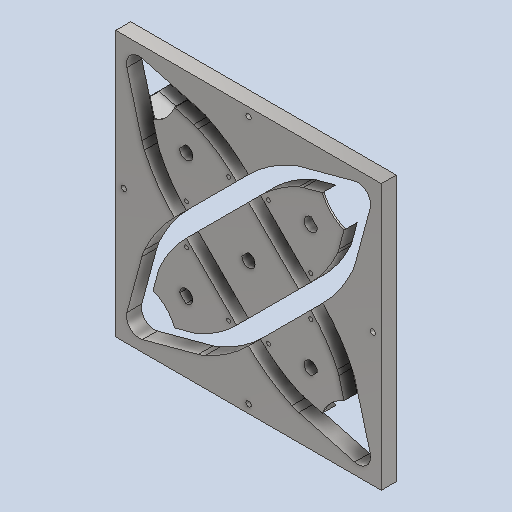
# Autodesk Inventor part: GuidePlateMetal
Saved by Autodesk Inventor 2022 (Build 260153000, 153)
## iProperties
Created: 2020-03-15
Part Number: GuidePlateMetal
Material: Generic
Document SubType Name: Modeling
Designer: elmar
Density: 1 g/cm^3
Appearance: Default
Author: elmar
Autodesk Inventor part; units mm, degrees
ref_plane "YZ Plane" through (0, 0, 0) normal (1, 0, 0) x (0, 1, 0)
ref_plane "XZ Plane" through (0, 0, 0) normal (0, 1, 0) x (-1, 0, 0)
sketch "Sketch41" plane through (0, 0, 0) normal (0, 0, 1) x (1, 0, 0)
  line L0 (80, -80) -> (-80, -80)
  line L1 (-80, -80) -> (-80, 80)
  line L2 (-80, 80) -> (80, 80)
  line L3 (80, 80) -> (80, -80)
  line L4 (80, -80) -> (-80, 80) construction
  line L5 (-80, -80) -> (80, 80) construction
  circle A0 centre (-37.5, 37.5) radius 37.5
  line L6 (0, -112) -> (0, 112) projected
  line L7 (-112, 0) -> (112, 0) projected
  circle A1 centre (-37.5, 37.5) radius 31.6165
  circle A2 centre (-37.5, 37.5) radius 21.4165
  circle A3 centre (37.5, -37.5) radius 31.6165
  circle A4 centre (37.5, -37.5) radius 21.4165
  line L8 (59.8562, -15.1438) -> (-15.1438, 59.8562)
  line L9 (52.6438, -22.3562) -> (-22.3562, 52.6438)
  line L10 (15.1438, -59.8562) -> (-59.8562, 15.1438)
  line L11 (22.3562, -52.6438) -> (-52.6438, 22.3562)
  circle A5 centre (-37.5, -37.5) radius 31.6165
  circle A6 centre (-37.5, -37.5) radius 21.4165
  circle A7 centre (37.5, 37.5) radius 31.6165
  circle A8 centre (37.5, 37.5) radius 21.4165
  line L12 (59.8562, 15.1438) -> (-15.1438, -59.8562)
  line L13 (52.6438, 22.3562) -> (-22.3562, -52.6438)
  line L14 (15.1438, 59.8562) -> (-59.8562, -15.1438)
  line L15 (22.3562, 52.6438) -> (-52.6438, -22.3562)
  line L16 (-37.5, 37.5) -> (-37.5, -37.5)
  circle A9 centre (-60.481, 60.481) radius 5
  line L17 (-49.8744, 49.8744) -> (-71.0876, 71.0876)
  arc A10 (-49.8744, 49.8744) -> (-71.0876, 71.0876) centre (-74.6231, 46.3388) ccw
  arc A11 (-71.0876, 71.0876) -> (-49.8744, 49.8744) centre (-46.3388, 74.6231) ccw
  arc A12 (-49.6403, 49.6403) -> (-71.3216, 71.3216) centre (-74.6231, 46.3388) ccw
  arc A13 (-71.3216, 71.3216) -> (-49.6403, 49.6403) centre (-46.3388, 74.6231) ccw
  line L18 (53.6853, -18.7098) -> (35.2271, 4.9396)
  circle A14 centre (44.4562, -6.8851) radius 5
  arc A15 (35.2271, 4.9396) -> (53.6853, -18.7098) centre (60.2225, 5.4203) ccw
  arc A16 (53.6853, -18.7098) -> (35.2271, 4.9396) centre (28.6899, -19.1906) ccw
  circle A17 centre (-37.5, 37.5) radius 17.5
  circle A18 centre (-37.5, 37.5) radius 7.5
  line L19 (-71.3216, 71.3216) -> (-49.6403, 49.6403)
  line L20 (-52.6438, 22.3562) -> (-59.8562, 15.1438)
  arc A19 (-62.7512, 26.1128) -> (-44.7125, 0) centre (17.6641, 62.3766) ccw
  arc A20 (-53.4529, 30.3059) -> (-37.5, 7.2125) centre (17.6641, 62.3766) ccw
  arc A21 (0, 44.7125) -> (-26.1128, 62.7512) centre (-62.3766, -17.6641) ccw
  arc A22 (-7.2125, 37.5) -> (-30.3059, 53.4529) centre (-62.3766, -17.6641) ccw
  line L21 (-37.5, 37.5) -> (-26.1128, 62.7512)
  circle A23 centre (-37.5, 37.5) radius 27.7
  circle A24 centre (-65.9013, 65.9013) radius 7.6655
  line L22 (-73.1417, 68.4185) -> (-44.18, 58.3498)
  line L23 (-73.5645, 66.0883) -> (-42.9116, 65.3403)
  line L24 (-73.038, 68.6991) -> (-44.4913, 57.5078)
  line L25 (-30.2936, 64.2462) -> (-63.9071, 73.3029)
  line L26 (-32.9472, 54.3974) -> (-44.4913, 57.5078)
  arc A25 (-60.0448, 43.663) -> (-44.4913, 57.5078) centre (-65.9013, 65.9013) ccw
  line L27 (-64.2462, 30.2936) -> (-73.3029, 63.9071)
  line L28 (-54.3974, 32.9472) -> (-57.5078, 44.4913)
  circle A26 centre (-37.5, 37.5) radius 4
  line L29 (-37.7505, 41.4921) -> (-41.4921, 37.7505)
  circle A27 centre (0, 0) radius 4
  line L30 (-0.2505, 3.9921) -> (-3.9921, 0.2505)
  point P0 (-37.5, 7.2125)
  point P1 (44.7125, 0)
  point P2 (-30.2875, 0)
  point P3 (-60.481, 60.481)
  dimension "d1039" = 35
  dimension "TrackWidth" = 10.2
  dimension "d715" = 160
  dimension "d718" = 75
  dimension "d721" = 10
  dimension "d722" = 30
  dimension "d723" = 0.2
  dimension "d1003" = 10
  dimension "d1004" = 30
  dimension "d1040" = 15
  dimension "d1487" = 8
  dimension "d1488" = 3
  constraints: 58 end point, 36 point on circle, 19 centre point, 17 point on line, 15 symmetric about line, 11 tangent, 9 coincident, 5 equal length, 5 horizontal, 5 parallel, 4 midpoint, 3 equal radius, 3 perpendicular, 1 concentric, 62 other
  measures "d715" distance of L1.end L2.end
  measures "d718" diameter of A0
  measures "d721" diameter of A9
  measures "d722" distance of L17.end L17.start
  measures "d723" radial gap between concentric circles of A10 A12
  measures "d1003" diameter of A14
  measures "d1004" distance of L18.start L18.end
  measures "d1040" diameter of A18
  measures "d1487" diameter of A26
  measures "d1488" distance from line of A0.centre L29
extrude "Extrusion39" add sketch "Sketch41" along normal blind 8
sketch "Sketch42" plane through (0, 0, 0) normal (0, 0, -1) x (-1, 0, 0)
  circle A0 centre (37.5, 37.5) radius 31.6165 projected
  circle A1 centre (37.5, 37.5) radius 21.4165 projected
  line L0 (-59.8562, -15.1438) -> (15.1438, 59.8562) projected
  line L1 (-52.6438, -22.3562) -> (22.3562, 52.6438) projected
  line L2 (-59.8562, 15.1438) -> (15.1438, -59.8562) projected
  line L3 (-15.1438, 59.8562) -> (59.8562, -15.1438) projected
  line L4 (-22.3562, -52.6438) -> (52.6438, 22.3562) projected
  line L5 (-15.1438, -59.8562) -> (59.8562, 15.1438) projected
  line L6 (-22.3562, 52.6438) -> (52.6438, -22.3562) projected
  arc A2 (44.7125, 0) -> (62.7512, 26.1128) centre (-17.6641, 62.3766) ccw projected
  arc A3 (37.5, 7.2125) -> (53.4529, 30.3059) centre (-17.6641, 62.3766) ccw projected
  arc A4 (26.1128, 62.7512) -> (0, 44.7125) centre (62.3766, -17.6641) ccw projected
  arc A5 (30.3059, 53.4529) -> (7.2125, 37.5) centre (62.3766, -17.6641) ccw projected
  line L7 (32.9472, 54.3974) -> (44.4913, 57.5078) projected
  arc A6 (44.4913, 57.5078) -> (60.0448, 43.663) centre (65.9013, 65.9013) ccw projected
  line L8 (54.3974, 32.9472) -> (57.5078, 44.4913) projected
  line L9 (30.2936, 64.2462) -> (63.9071, 73.3029) projected
  line L10 (64.2462, 30.2936) -> (73.3029, 63.9071) projected
  circle A7 centre (65.9013, 65.9013) radius 7.6655 projected
  circle A8 centre (37.5, 37.5) radius 17.5 projected
  circle A9 centre (37.5, 37.5) radius 27.7 projected
  point P0 (0, 0)
  point P1 (-44.7125, 0)
  point P2 (-37.5, -7.2125)
  point P3 (37.5, 7.2125)
  point P4 (44.7125, 0)
  point P5 (5.9103, 36.1978)
  point P6 (38.8022, 5.9103)
  point P7 (36.1978, 5.9103)
  point P8 (-7.2125, -37.5)
  point P9 (0, -44.7125)
  point P10 (7.2125, 37.5)
  point P11 (0, 44.7125)
  point P12 (5.9103, 38.8022)
  point P13 (60.5726, 60.5726)
  point P14 (10.2177, 53.4775)
  point P15 (53.4775, 10.2177)
  point P16 (-7.2125, 37.5)
  point P17 (30.2875, 0)
  point P18 (44.7125, 0)
  point P19 (47.9316, 51.551)
  point P20 (51.551, 47.9316)
  point P21 (45.0106, 68.2115)
  point P22 (68.2115, 45.0106)
  point P23 (0, 44.7125)
extrude "Extrusion40" cut sketch "Sketch42" against normal through all contours A2 L3 A0 | A0 L3 L4 A9 A2 | L10 A9 L9 A0 | A0 L9 A7 L10 | A9 L4 A1 L1 | A7 | L4 L6 A0 | A0 L1 L3 A9 L4 | A3 A9 L4 | A9 A3 A1 L4 | L6 L1 A0 | A9 L3 | A1 A3 A8 L8 A6 | A4 A9 L1 L3 A0 | A0 L3 A4 | L3 A0 L1 L6 L0 | A0 L3 L1 | A9 A5 L1 | L1 A1 A5 A9 | A1 A6 A8 L7 A5 | A6 A8 picked at (49.9917, 49.5888)
ref_plane "Work Plane2" through (0, 0, 7) normal (0, 0, 1) x (1, 0, 0)
extrude "Extrusion73" cut sketch "Sketch41" along normal through all contours A26 L16 L21 | L21 L16 A26 L29
extrude "Extrusion74" cut sketch "Sketch41" along normal through all contours A27 L7 L6 | L6 L7 A27 | L7 A27 L30 L6 | L6 A27 L7
ref_plane "Work Plane3" through (-80, 80, 0) normal (0.7071068, 0.7071068, 0) x (0, 0, 1)
pattern_circular "Circular Pattern6" count 4 over 360 about axis through (0, 0, -10) along (0, 0, 1) of "Extrusion40", "Extrusion73"
ref_plane "Work Plane6" through (-37.5, 7.2125, 7) normal (0, 0, 1) x (0.7071068, -0.7071068, 0)
sketch "Sketch75" plane through (0, 0, 7) normal (0, 0, -1) x (-1, 0, 0)
  arc A0 (37.5, 7.2125) -> (53.4529, 30.3059) centre (-17.6641, 62.3766) ccw projected
  arc A1 (53.4529, 30.3059) -> (54.3974, 32.9472) centre (37.5, 37.5) ccw projected
  line L0 (54.3974, 32.9472) -> (57.5078, 44.4913) projected
  arc A2 (44.4913, 57.5078) -> (57.5078, 44.4913) centre (65.9013, 65.9013) ccw projected
  line L1 (44.4913, 57.5078) -> (32.9472, 54.3974) projected
  arc A3 (32.9472, 54.3974) -> (30.3059, 53.4529) centre (37.5, 37.5) ccw projected
  arc A4 (30.3059, 53.4529) -> (7.2125, 37.5) centre (62.3766, -17.6641) ccw projected
  line L2 (7.2125, 37.5) -> (37.5, 7.2125) projected
  line L3 (-112, -112) -> (112, 112) projected
  line L4 (14.4366, 31.6901) -> (37.2742, 54.5276)
  line L5 (37.2742, 54.5276) -> (43.0737, 56.0902)
  line L6 (43.0737, 56.0902) -> (44.4913, 57.5078)
  line L7 (37.5, 37.5) -> (22.3562, 22.3562) construction
  line L8 (37.5, 7.2125) -> (7.2125, 37.5) projected
  line L9 (33.9645, 41.0355) -> (18.8207, 25.8918)
  line L10 (25.8918, 18.8207) -> (41.0355, 33.9645)
  arc A5 (41.0355, 33.9645) -> (33.9645, 41.0355) centre (37.5, 37.5) ccw
  arc A6 (18.8207, 25.8918) -> (25.8918, 18.8207) centre (22.3562, 22.3562) ccw
  line L11 (14.4366, 31.6901) -> (19.5278, 26.5989)
  arc A7 (44.4913, 57.5078) -> (57.5078, 44.4913) centre (65.9013, 65.9013) ccw projected
  line L12 (31.6901, 14.4366) -> (54.5276, 37.2742)
  line L13 (54.5276, 37.2742) -> (56.0902, 43.0737)
  line L14 (56.0902, 43.0737) -> (57.5078, 44.4913)
  line L15 (31.6901, 14.4366) -> (26.5989, 19.5278)
  point P0 (0, 0)
  point P1 (57.5078, 44.4913)
  dimension "d1056" = 5
  dimension "d1057" = 1
  dimension "SpringTipGuideWidth" = 7.2
  dimension "d1059" = 1
  constraints: 24 end point, 5 symmetric about line, 4 parallel, 4 point on circle, 4 tangent, 3 point on line, 2 centre point, 1 midpoint, 1 perpendicular
  measures "d1056" radius of A5
  measures "d1057" distance between parallel lines of L5 L1
  measures "SpringTipGuideWidth" distance of L4.start L11.end
  measures "d1059" distance between parallel lines of L8 L11
extrude "Extrusion50" cut sketch "Sketch75" along normal up to surface (7 mm away) contours L10 A5 L3 A2 L14 L13 L12 L15 | A5 L9 L11 L4 L5 L6 A2 L3
sketch "Sketch79" plane through (0, 0, 7) normal (0, 0, -1) x (-1, 0, 0)
  line L0 (-30.2875, 0) -> (0, 30.2875) projected
  line L1 (0, 30.2875) -> (30.2875, 0) projected
  line L2 (30.2875, 0) -> (0, -30.2875) projected
  line L3 (0, -30.2875) -> (-30.2875, 0) projected
  line L4 (54.3974, -32.9472) -> (57.5078, -44.4913) projected
  arc A0 (57.5078, -44.4913) -> (44.4913, -57.5078) centre (65.9013, -65.9013) ccw projected
  line L5 (44.4913, -57.5078) -> (32.9472, -54.3974) projected
  arc A1 (30.3059, -53.4529) -> (32.9472, -54.3974) centre (37.5, -37.5) ccw projected
  arc A2 (7.2125, -37.5) -> (30.3059, -53.4529) centre (62.3766, 17.6641) ccw projected
  line L6 (7.2125, -37.5) -> (37.5, -7.2125) projected
  arc A3 (53.4529, -30.3059) -> (37.5, -7.2125) centre (-17.6641, -62.3766) ccw projected
  arc A4 (54.3974, -32.9472) -> (53.4529, -30.3059) centre (37.5, -37.5) ccw projected
  arc A5 (-44.4913, -57.5078) -> (-57.5078, -44.4913) centre (-65.9013, -65.9013) ccw projected
  line L7 (-57.5078, -44.4913) -> (-54.3974, -32.9472) projected
  arc A6 (-53.4529, -30.3059) -> (-54.3974, -32.9472) centre (-37.5, -37.5) ccw projected
  arc A7 (-37.5, -7.2125) -> (-53.4529, -30.3059) centre (17.6641, -62.3766) ccw projected
  line L8 (-37.5, -7.2125) -> (-7.2125, -37.5) projected
  arc A8 (-30.3059, -53.4529) -> (-7.2125, -37.5) centre (-62.3766, 17.6641) ccw projected
  arc A9 (-32.9472, -54.3974) -> (-30.3059, -53.4529) centre (-37.5, -37.5) ccw projected
  line L9 (-32.9472, -54.3974) -> (-44.4913, -57.5078) projected
  line L10 (56.0902, 43.0737) -> (57.5078, 44.4913) projected
  arc A10 (44.4913, 57.5078) -> (57.5078, 44.4913) centre (65.9013, 65.9013) ccw projected
  line L11 (44.4913, 57.5078) -> (43.0737, 56.0902) projected
  line L12 (43.0737, 56.0902) -> (37.2742, 54.5276) projected
  line L13 (37.2742, 54.5276) -> (14.4366, 31.6901) projected
  line L14 (14.4366, 31.6901) -> (19.5278, 26.5989) projected
  line L15 (19.5278, 26.5989) -> (33.9645, 41.0355) projected
  arc A11 (41.0355, 33.9645) -> (33.9645, 41.0355) centre (37.5, 37.5) ccw projected
  line L16 (41.0355, 33.9645) -> (26.5989, 19.5278) projected
  line L17 (26.5989, 19.5278) -> (31.6901, 14.4366) projected
  line L18 (31.6901, 14.4366) -> (54.5276, 37.2742) projected
  line L19 (54.5276, 37.2742) -> (56.0902, 43.0737) projected
  line L20 (57.5078, 44.4913) -> (54.3974, 32.9472) projected
  arc A12 (53.4529, 30.3059) -> (54.3974, 32.9472) centre (37.5, 37.5) ccw projected
  arc A13 (37.5, 7.2125) -> (53.4529, 30.3059) centre (-17.6641, 62.3766) ccw projected
  line L21 (37.5, 7.2125) -> (7.2125, 37.5) projected
  arc A14 (30.3059, 53.4529) -> (7.2125, 37.5) centre (62.3766, -17.6641) ccw projected
  arc A15 (32.9472, 54.3974) -> (30.3059, 53.4529) centre (37.5, 37.5) ccw projected
  line L22 (32.9472, 54.3974) -> (44.4913, 57.5078) projected
  arc A16 (0, 44.7125) -> (-26.1128, 62.7512) centre (-62.3766, -17.6641) ccw projected
  arc A17 (-26.1128, 62.7512) -> (-30.2936, 64.2462) centre (-37.5, 37.5) ccw projected
  line L23 (-30.2936, 64.2462) -> (-63.9071, 73.3029) projected
  arc A18 (-63.9071, 73.3029) -> (-73.3029, 63.9071) centre (-65.9013, 65.9013) ccw projected
  line L24 (-73.3029, 63.9071) -> (-64.2462, 30.2936) projected
  arc A19 (-64.2462, 30.2936) -> (-62.7512, 26.1128) centre (-37.5, 37.5) ccw projected
  arc A20 (-62.7512, 26.1128) -> (-44.7125, 0) centre (17.6641, 62.3766) ccw projected
  arc A21 (-44.7125, 0) -> (-62.7512, -26.1128) centre (17.6641, -62.3766) ccw projected
  arc A22 (-62.7512, -26.1128) -> (-64.2462, -30.2936) centre (-37.5, -37.5) ccw projected
  line L25 (-64.2462, -30.2936) -> (-73.3029, -63.9071) projected
  arc A23 (-73.3029, -63.9071) -> (-63.9071, -73.3029) centre (-65.9013, -65.9013) ccw projected
  line L26 (-63.9071, -73.3029) -> (-30.2936, -64.2462) projected
  arc A24 (-30.2936, -64.2462) -> (-26.1128, -62.7512) centre (-37.5, -37.5) ccw projected
  arc A25 (-26.1128, -62.7512) -> (0, -44.7125) centre (-62.3766, 17.6641) ccw projected
  arc A26 (0, -44.7125) -> (26.1128, -62.7512) centre (62.3766, 17.6641) ccw projected
  arc A27 (26.1128, -62.7512) -> (30.2936, -64.2462) centre (37.5, -37.5) ccw projected
  line L27 (30.2936, -64.2462) -> (63.9071, -73.3029) projected
  arc A28 (63.9071, -73.3029) -> (73.3029, -63.9071) centre (65.9013, -65.9013) ccw projected
  line L28 (73.3029, -63.9071) -> (64.2462, -30.2936) projected
  arc A29 (64.2462, -30.2936) -> (62.7512, -26.1128) centre (37.5, -37.5) ccw projected
  arc A30 (62.7512, -26.1128) -> (44.7125, 0) centre (-17.6641, -62.3766) ccw projected
  arc A31 (44.7125, 0) -> (62.7512, 26.1128) centre (-17.6641, 62.3766) ccw projected
  arc A32 (62.7512, 26.1128) -> (64.2462, 30.2936) centre (37.5, 37.5) ccw projected
  line L29 (64.2462, 30.2936) -> (73.3029, 63.9071) projected
  arc A33 (73.3029, 63.9071) -> (63.9071, 73.3029) centre (65.9013, 65.9013) ccw projected
  line L30 (63.9071, 73.3029) -> (30.2936, 64.2462) projected
  arc A34 (30.2936, 64.2462) -> (26.1128, 62.7512) centre (37.5, 37.5) ccw projected
  arc A35 (26.1128, 62.7512) -> (0, 44.7125) centre (62.3766, -17.6641) ccw projected
  line L31 (80, 80) -> (80, -80) projected
  line L32 (80, -80) -> (-80, -80) projected
  line L33 (-80, -80) -> (-80, 80) projected
  line L34 (-80, 80) -> (80, 80) projected
  line L35 (-54.3974, 32.9472) -> (-57.5078, 44.4913) projected
  arc A36 (-57.5078, 44.4913) -> (-44.4913, 57.5078) centre (-65.9013, 65.9013) ccw projected
  line L36 (-44.4913, 57.5078) -> (-32.9472, 54.3974) projected
  arc A37 (-30.3059, 53.4529) -> (-32.9472, 54.3974) centre (-37.5, 37.5) ccw projected
  arc A38 (-7.2125, 37.5) -> (-30.3059, 53.4529) centre (-62.3766, -17.6641) ccw projected
  line L37 (-7.2125, 37.5) -> (-37.5, 7.2125) projected
  arc A39 (-53.4529, 30.3059) -> (-37.5, 7.2125) centre (17.6641, 62.3766) ccw projected
  arc A40 (-54.3974, 32.9472) -> (-53.4529, 30.3059) centre (-37.5, 37.5) ccw projected
  line L38 (57.5599, 44.6849) -> (56.0006, 43.1255)
  line L39 (56.0006, 43.1255) -> (54.438, 37.326)
  line L40 (54.438, 37.326) -> (31.6901, 14.5781)
  line L41 (31.6901, 14.5781) -> (26.7403, 19.5278)
  line L42 (26.7403, 19.5278) -> (41.1062, 33.8938)
  arc A41 (41.1062, 33.8938) -> (33.8938, 41.1062) centre (37.5, 37.5) ccw
  line L43 (33.8938, 41.1062) -> (19.5278, 26.7403)
  line L44 (19.5278, 26.7403) -> (14.5781, 31.6901)
  line L45 (14.5781, 31.6901) -> (37.326, 54.438)
  line L46 (37.326, 54.438) -> (43.1255, 56.0006)
  line L47 (43.1255, 56.0006) -> (44.6849, 57.5599)
  line L48 (23.0414, 40.1534) -> (27.9912, 35.2037)
  line L49 (44.6849, 57.5599) -> (55.0263, 60.3463)
  line L50 (44.4913, 57.5078) -> (32.9472, 54.3974) projected
  line L51 (38.7997, 55.9117) -> (37.4678, 54.5797)
  line L52 (43.0737, 56.0902) -> (43.2672, 56.1423)
  line L53 (37.2742, 54.5276) -> (43.0737, 56.0902) projected
  line L54 (-112, -112) -> (112, 112) projected
  arc A42 (44.4913, 57.5078) -> (57.5078, 44.4913) centre (65.9013, 65.9013) ccw projected
  line L55 (40.1534, 23.0414) -> (35.2037, 27.9912)
  line L56 (57.5599, 44.6849) -> (60.3463, 55.0263)
  line L57 (55.9117, 38.7997) -> (54.5797, 37.4678)
  line L58 (56.0902, 43.0737) -> (56.1423, 43.2672)
  line L59 (33.8938, 41.1062) -> (41.7207, 48.9332)
  arc A43 (48.9332, 48.9332) -> (41.7207, 48.9332) centre (45.327, 45.327) ccw
  line L60 (41.1062, 33.8938) -> (48.9332, 41.7207)
  arc A44 (48.9332, 41.7207) -> (48.9332, 48.9332) centre (45.327, 45.327) ccw
  arc A45 (55.0263, 60.3463) -> (60.3463, 55.0263) centre (73.7283, 73.7283) ccw
  arc A46 (-41.4921, 37.7505) -> (-37.7505, 41.4921) centre (-37.5, 37.5) ccw projected
  line L61 (-37.7505, 41.4921) -> (-41.4921, 37.7505) projected
  line L62 (3.9921, 0.2505) -> (0.2505, 3.9921) projected
  arc A47 (0.2505, 3.9921) -> (3.9921, 0.2505) centre (0, 0) ccw projected
  line L63 (37.7505, -41.4921) -> (41.4921, -37.7505) projected
  arc A48 (41.4921, -37.7505) -> (37.7505, -41.4921) centre (37.5, -37.5) ccw projected
  arc A49 (37.7505, 41.4921) -> (41.4921, 37.7505) centre (37.5, 37.5) ccw projected
  line L64 (41.4921, 37.7505) -> (37.7505, 41.4921) projected
  line L65 (-41.4921, -37.7505) -> (-37.7505, -41.4921) projected
  arc A50 (-37.7505, -41.4921) -> (-41.4921, -37.7505) centre (-37.5, -37.5) ccw projected
  point P0 (49.6403, 49.6403)
  point P1 (57.4673, 57.4673)
  point P2 (35.2037, 27.9912)
  point P3 (41.1062, 41.1062)
  point P4 (56.1423, 43.2672)
  point P5 (55.0639, 39.6489)
  point P6 (54.5797, 37.4678)
  point P7 (39.6489, 55.0639)
  dimension "d1077" = 0.1
  dimension "d1078" = 12.069
  dimension "d1079" = 11.069
  dimension "d1083" = 1
  dimension "SpringMaxCompression" = 11.069
  constraints: 40 end point, 11 point on circle, 4 centre point, 4 collinear, 4 point on line, 2 tangent, 1 coincident, 1 concentric, 1 equal radius, 1 parallel, 1 perpendicular, 25 other
  measures "d1077" distance between parallel lines of L45 L13
  measures "d1078" distance between parallel lines of L48 L14
  measures "d1079" distance of point (57.467, 57.467) point (49.64, 49.64)
  measures "d1083" distance of point (49.64, 49.64) A43.start
  measures "SpringMaxCompression" distance of point (48.933, 48.933) point (41.106, 41.106)
extrude "Extrusion52" add sketch "Sketch79" along normal blind 7 separate body contours L38 L39 L40 L55 L42 L60 A44 L54 A10 | A10 L54 A45 L56 L38 | L47 L49 A45 L54 A10 | A10 L54 A43 L59 L43 L48 L45 L46 L47
sketch "Sketch80" plane through (-27.9912, 35.2037, 7) normal (0.7071068, -0.7071068, 0) x (-0.7071068, -0.7071068, 0)
  line L0 (-7, 7) -> (0, 0)
  line L1 (-7, 0) -> (-7, 7) projected
  line L2 (-7, 7) -> (0, 7) projected
  line L3 (0, 7) -> (0, 0) projected
  line L4 (0, 0) -> (-7, 0) projected
  line L5 (10.2, 0) -> (10.2, 7) projected
  line L6 (10.2, 7) -> (17.2, 7) projected
  line L7 (17.2, 7) -> (17.2, 0) projected
  line L8 (17.2, 0) -> (10.2, 0) projected
  circle A0 centre (-3.5, 3.5) radius 2.75
  line L9 (25.414, -1) -> (-15.214, -1) projected
  line L10 (-15.214, -1) -> (-15.214, 7) projected
  line L11 (-15.214, 7) -> (-7.1, 7) projected
  line L12 (-7.1, 7) -> (-7.1, 0) projected
  line L13 (-7.1, 0) -> (0.1, 0) projected
  line L14 (0.1, 0) -> (0.1, 7) projected
  line L15 (0.1, 7) -> (10.1, 7) projected
  line L16 (10.1, 7) -> (10.1, 0) projected
  line L17 (10.1, 0) -> (17.3, 0) projected
  line L18 (17.3, 0) -> (17.3, 7) projected
  line L19 (17.3, 7) -> (25.414, 7) projected
  line L20 (25.414, 7) -> (25.414, -1) projected
  line L21 (-63.3516, 7) -> (-25.543, 7) projected
  line L22 (-25.543, 7) -> (-25.543, -1) projected
  line L23 (-25.543, -1) -> (-63.3516, -1) projected
  line L24 (-63.3516, -1) -> (-63.3516, 7) projected
  line L25 (35.743, 7) -> (73.5516, 7) projected
  line L26 (73.5516, 7) -> (73.5516, -1) projected
  line L27 (73.5516, -1) -> (35.743, -1) projected
  line L28 (35.743, -1) -> (35.743, 7) projected
  point P0 (5.1, 7)
  dimension "d1092" = 5.5
  constraints: 2 end point, 1 centre point, 1 coincident, 1 midpoint
  measures "d1092" diameter of A0
sketch "Sketch81" plane through (0, 0, 0) normal (0, 0, 1) x (1, 0, 0)
  line L0 (-44.6849, 57.5599) -> (-43.1255, 56.0006) projected
  line L1 (-43.1255, 56.0006) -> (-37.326, 54.438) projected
  line L2 (-37.326, 54.438) -> (-23.0414, 40.1534) projected
  line L3 (-23.0414, 40.1534) -> (-27.9912, 35.2037) projected
  line L4 (-27.9912, 35.2037) -> (-41.7207, 48.9332) projected
  arc A0 (-41.7207, 48.9332) -> (-48.9332, 41.7207) centre (-45.327, 45.327) ccw projected
  line L5 (-48.9332, 41.7207) -> (-35.2037, 27.9912) projected
  line L6 (-35.2037, 27.9912) -> (-40.1534, 23.0414) projected
  line L7 (-40.1534, 23.0414) -> (-54.438, 37.326) projected
  line L8 (-54.438, 37.326) -> (-56.0006, 43.1255) projected
  line L9 (-56.0006, 43.1255) -> (-57.5599, 44.6849) projected
  line L10 (-57.5599, 44.6849) -> (-60.3463, 55.0263) projected
  line L11 (-55.0263, 60.3463) -> (-44.6849, 57.5599) projected
  line L12 (-25.5163, 37.6785) -> (-39.8009, 51.9631)
  arc A1 (-60.3463, 55.0263) -> (-55.0263, 60.3463) centre (-73.7283, 73.7283) ccw projected
  point P0 (0, 0)
  dimension "SpringTipHoleDepth" = 20.2014
  constraints: 3 end point, 1 midpoint, 1 parallel, 1 perpendicular
  measures "SpringTipHoleDepth" distance of L12.start L12.end
sweep "Sweep1" cut profiles "Sketch80" path "Sketch81" bodies 2 path curves L12 contours A0 L0 | L0 A0
mirror "Mirror7" about plane through (-80, 80, 0) normal (0.7071068, 0.7071068, 0) of "Sweep1" bodies 2
sketch "Sketch83" plane through (-31.6901, 14.4366, 0) normal (-0.7071068, 0.7071068, 0) x (-0.7071068, -0.7071068, 0)
  circle A0 centre (-3.6, 3.5) radius 2.75 projected
  circle A1 centre (-3.6, 3.5) radius 1.25
  point P0 (-12.2, 0)
  dimension "d1103" = 2.5
  constraints: 1 centre point, 1 coincident
  measures "d1103" diameter of A1
extrude "Extrusion54" add sketch "Sketch83" along normal blind 1 contours A1 bodies 1
mirror "Mirror8" about plane through (-80, 80, 0) normal (0.7071068, 0.7071068, 0) of "Extrusion54" bodies 1
sketch "Sketch84" plane through (-37.5, 7.2125, 0) normal (0, 0, -1) x (-0.7071068, 0.7071068, 0)
  arc A0 (21.4165, 16.4165) -> (21.4165, 26.4165) centre (21.4165, 21.4165) ccw projected
  line L0 (1, 16.4165) -> (21.4165, 16.4165) projected
  circle A1 centre (21.4165, 21.4165) radius 5
  line L1 (24.4165, 24.0623) -> (24.4165, 18.7708) projected
  arc A2 (24.4165, 24.0623) -> (24.4165, 18.7708) centre (21.4165, 21.4165) ccw projected
  point P0 (-31.6165, 21.4165)
  point P1 (21.4165, 26.4165)
  constraints: 1 coincident, 3 other
extrude "Extrusion55" add sketch "Sketch84" along normal blind 1 bodies 1
pattern_circular "Circular Pattern7" count 4 over 360 about axis through (0, 0, -10) along (0, 0, 1) of "Extrusion50", "Extrusion54", "Mirror8", "Extrusion55" bodies 1
sketch "Sketch101" plane through (0, 0, 0) normal (0, 0, -1) x (-1, 0, 0)
  line L0 (0, 30.2875) -> (-30.2875, 0) projected
  line L1 (-30.2875, 0) -> (0, -30.2875) projected
  line L2 (0, -30.2875) -> (30.2875, 0) projected
  line L3 (30.2875, 0) -> (0, 30.2875) projected
  arc A0 (0, 44.7125) -> (-26.1128, 62.7512) centre (-62.3766, -17.6641) ccw projected
  arc A1 (26.1128, 62.7512) -> (0, 44.7125) centre (62.3766, -17.6641) ccw projected
  arc A2 (30.2936, 64.2462) -> (26.1128, 62.7512) centre (37.5, 37.5) ccw projected
  line L4 (30.2936, 64.2462) -> (63.9071, 73.3029) projected
  arc A3 (73.3029, 63.9071) -> (63.9071, 73.3029) centre (65.9013, 65.9013) ccw projected
  line L5 (73.3029, 63.9071) -> (64.2462, 30.2936) projected
  arc A4 (62.7512, 26.1128) -> (64.2462, 30.2936) centre (37.5, 37.5) ccw projected
  arc A5 (44.7125, 0) -> (62.7512, 26.1128) centre (-17.6641, 62.3766) ccw projected
  arc A6 (62.7512, -26.1128) -> (44.7125, 0) centre (-17.6641, -62.3766) ccw projected
  arc A7 (64.2462, -30.2936) -> (62.7512, -26.1128) centre (37.5, -37.5) ccw projected
  line L6 (64.2462, -30.2936) -> (73.3029, -63.9071) projected
  arc A8 (63.9071, -73.3029) -> (73.3029, -63.9071) centre (65.9013, -65.9013) ccw projected
  line L7 (63.9071, -73.3029) -> (30.2936, -64.2462) projected
  arc A9 (26.1128, -62.7512) -> (30.2936, -64.2462) centre (37.5, -37.5) ccw projected
  arc A10 (0, -44.7125) -> (26.1128, -62.7512) centre (62.3766, 17.6641) ccw projected
  arc A11 (-26.1128, -62.7512) -> (0, -44.7125) centre (-62.3766, 17.6641) ccw projected
  arc A12 (-30.2936, -64.2462) -> (-26.1128, -62.7512) centre (-37.5, -37.5) ccw projected
  line L8 (-30.2936, -64.2462) -> (-63.9071, -73.3029) projected
  arc A13 (-73.3029, -63.9071) -> (-63.9071, -73.3029) centre (-65.9013, -65.9013) ccw projected
  line L9 (-73.3029, -63.9071) -> (-64.2462, -30.2936) projected
  arc A14 (-62.7512, -26.1128) -> (-64.2462, -30.2936) centre (-37.5, -37.5) ccw projected
  arc A15 (-44.7125, 0) -> (-62.7512, -26.1128) centre (17.6641, -62.3766) ccw projected
  arc A16 (-62.7512, 26.1128) -> (-44.7125, 0) centre (17.6641, 62.3766) ccw projected
  arc A17 (-64.2462, 30.2936) -> (-62.7512, 26.1128) centre (-37.5, 37.5) ccw projected
  line L10 (-64.2462, 30.2936) -> (-73.3029, 63.9071) projected
  arc A18 (-63.9071, 73.3029) -> (-73.3029, 63.9071) centre (-65.9013, 65.9013) ccw projected
  line L11 (-63.9071, 73.3029) -> (-30.2936, 64.2462) projected
  arc A19 (-26.1128, 62.7512) -> (-30.2936, 64.2462) centre (-37.5, 37.5) ccw projected
  line L12 (80, -80) -> (-80, -80) projected
  line L13 (80, 80) -> (80, -80) projected
  line L14 (-80, 80) -> (80, 80) projected
  line L15 (-80, -80) -> (-80, 80) projected
  arc A20 (0.2505, 3.9921) -> (3.9921, 0.2505) centre (0, 0) ccw projected
  line L16 (0.2505, 3.9921) -> (3.9921, 0.2505) projected
extrude "Extrusion60" add sketch "Sketch101" along normal blind 1 bodies 1
sketch "Sketch43" plane through (0, 0, -1) normal (0, 0, 1) x (1, 0, 0)
  line L0 (-75, -75) -> (75, -75)
  line L1 (75, -75) -> (75, 75)
  line L2 (75, 75) -> (-75, 75)
  line L3 (-75, 75) -> (-75, -75)
  line L4 (-75, -75) -> (75, 75) construction
  line L5 (75, -75) -> (-75, 75) construction
  line L6 (-80, 80) -> (80, 80) projected
  point P0 (0, 0)
  point P1 (0, 75)
  point P2 (-75, 0)
  point P3 (0, -75)
  point P4 (75, 0)
  point P5 (-80, -80)
  point P6 (80, -80)
  dimension "d1250" = 5
  constraints: 12 end point, 6 midpoint, 3 point on line, 2 parallel, 2 perpendicular, 1 horizontal
  measures "d1250" distance between parallel lines of L2 L6
hole "Hole6" at (0, 75, -1) at (-75, 0, -1) at (0, -75, -1) at (75, 0, -1) direction (0, 0, 1) diameter 3.2 end through all countersink diameter 6.3 countersink angle 90 bodies 1
sketch "Sketch96" plane through (0, 0, 0) normal (0, 0, -1) x (-1, 0, 0)
  line L0 (37.5, -7.2125) -> (7.2125, -37.5) projected
  arc A0 (53.4529, -30.3059) -> (37.5, -7.2125) centre (-17.6641, -62.3766) ccw projected
  arc A1 (54.3974, -32.9472) -> (53.4529, -30.3059) centre (37.5, -37.5) ccw projected
  line L1 (57.5078, -44.4913) -> (54.3974, -32.9472) projected
  arc A2 (57.5078, -44.4913) -> (44.4913, -57.5078) centre (65.9013, -65.9013) ccw projected
  line L2 (32.9472, -54.3974) -> (44.4913, -57.5078) projected
  arc A3 (30.3059, -53.4529) -> (32.9472, -54.3974) centre (37.5, -37.5) ccw projected
  arc A4 (7.2125, -37.5) -> (30.3059, -53.4529) centre (62.3766, 17.6641) ccw projected
  circle A5 centre (37.5, -37.5) radius 5 projected
  point P0 (0, 0)
extrude "Extrusion57" add sketch "Sketch96" along normal blind 1 separate body
sketch "Sketch99" plane through (0, 0, -1) normal (0, 0, -1) x (-1, 0, 0)
  line L0 (37.5, -7.2125) -> (7.2125, -37.5) projected
  arc A0 (53.4529, -30.3059) -> (37.5, -7.2125) centre (-17.6641, -62.3766) ccw projected
  arc A1 (7.2125, -37.5) -> (30.3059, -53.4529) centre (62.3766, 17.6641) ccw projected
  circle A2 centre (37.4468, -12.0033) radius 3.35
  circle A3 centre (12.0033, -37.4468) radius 3.35
  point P0 (0, 0)
  dimension "d1222" = 6.7
  dimension "d1482" = 2
  dimension "d1484" = 4
  dimension "d1485" = 2
  constraints: 4 tangent, 2 centre point, 1 equal radius
  measures "d1222" diameter of A2
hole "Hole11" at (-12.0033, -37.4468, -1) at (-37.4468, -12.0033, -1) direction (0, 0, 1) diameter 2.459 end through all countersink diameter 7 countersink angle 90 bodies 1
pattern_circular "Circular Pattern15" count 4 over 360 about axis through (0, 0, -10) along (0, 0, 1) of "Hole11" bodies 1 3
hole "Hole15" at (-37.4468, -12.0033, -1) at (-12.0033, -37.4468, -1) direction (0, 0, 1) diameter 3.2 end through all countersink diameter 7 countersink angle 90 bodies 3
sketch "Sketch132" plane through (0, 0, 0) normal (0, 0, -1) x (-1, 0, 0)
  line L0 (16.9008, 39.8111) -> (29.1532, 52.0634) projected
  arc A0 (30.047, 52.5803) -> (29.1532, 52.0634) centre (30.5674, 50.6492) ccw projected
  line L1 (30.047, 52.5803) -> (43.0737, 56.0902) projected
  line L2 (14.5583, 32.0946) -> (36.887, 54.4233)
  line L3 (37.326, 54.438) -> (23.0414, 40.1534) projected
  line L4 (14.5583, 32.0946) -> (16.4013, 38.9345)
  arc A1 (16.9182, 39.8284) -> (16.4013, 38.9345) centre (18.3324, 38.4142) ccw
  line L5 (14.5871, 32.2484) -> (16.3839, 38.9172) projected
  arc A2 (16.9008, 39.8111) -> (16.3839, 38.9172) centre (18.315, 38.3969) ccw projected
  arc A3 (14.5871, 32.2484) -> (14.8456, 31.2812) centre (15.5527, 31.9883) ccw projected
  point P0 (0, 0)
  point P1 (37.2742, 54.5276)
  point P2 (15.1438, 32.3972)
  dimension "d1493" = 0.3
  constraints: 3 midpoint, 2 end point, 1 coincident, 1 point on line, 1 vertical alignment, 2 other
  measures "d1493" distance between parallel lines of L3 L2
sketch "Sketch134" plane through (-23.4768, 49.9596, 3.5) normal (0.7071068, 0.7071068, 0) x (0, 0, 1)
  point P0 (-3.5, 51.9273)
  point P1 (0, 3.15)
  point P2 (0, 3.15)
  constraints: 1 coincident
equation "\"GearShaftDiameter\" = 8"
equation "\"TrackClearance\" = 0.2"
equation "\"d903\" = 55deg"
equation "\"Sketch59_Pitch\" = 1.25"
equation "\"d921\" = 55deg"
equation "\"Sketch61_Pitch\" = 1.25"
equation "\"d939\" = 55deg"
equation "\"Sketch63_Pitch\" = 1.25"
equation "\"d957\" = 55deg"
equation "\"Sketch65_Pitch\" = 1.25"
equation "\"d975\" = 55deg"
equation "\"Sketch67_Pitch\" = 1.25"
equation "\"d1117\" = 55deg"
equation "\"Sketch85_Pitch\" = 1.25"
equation "\"d1140\" = 55deg"
equation "\"Sketch87_Pitch\" = 1.25"
equation "\"d1160\" = 55deg"
equation "\"Sketch89_Pitch\" = 1.25"
equation "\"d1180\" = 55deg"
equation "\"Sketch91_Pitch\" = 1.25"
equation "\"d1202\" = 55deg"
equation "\"Sketch94_Pitch\" = 1.25"
equation "\"d1239\" = 55deg"
equation "\"Sketch102_Pitch\" = 1.25"
equation "\"d1269\" = 55deg"
equation "\"Sketch106_Pitch\" = 0.6"
equation "\"d1287\" = 55deg"
equation "\"Sketch108_Pitch\" = 0.6"
equation "\"d1320\" = 55deg"
equation "\"Sketch110_Pitch\" = 0.5"
equation "\"d1338\" = 55deg"
equation "\"Sketch112_Pitch\" = 0.5"
equation "\"d1356\" = 55deg"
equation "\"Sketch114_Pitch\" = 0.5"
equation "\"d1374\" = 55deg"
equation "\"Sketch116_Pitch\" = 0.5"
equation "\"d1392\" = 55deg"
equation "\"Sketch118_Pitch\" = 0.5"
equation "\"d1410\" = 55deg"
equation "\"Sketch120_Pitch\" = 0.5"
body "Srf5"
